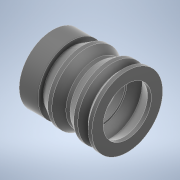
# Autodesk Inventor part: Daemper_TPU_Z2
Saved by Autodesk Inventor 2021 (Build 250183000, 183)
## iProperties
Created: 2022-06-20
Part Number: Daemper_TPU_Z2
Material: Thermoplastisches Harz
Document SubType Name: Modeling
Designer: Timo
Density: 1.28 g/cm^3
Appearance: Glatt - Schwarz
Mass: 1.13349 g
Surface Area: 19.2466 cm^2
Volume: 0.885539 cm^3
Author: Timo
Autodesk Inventor part; units mm, degrees
ref_plane "YZ Plane" through (0, 0, 0) normal (1, 0, 0) x (0, 1, 0)
ref_plane "XZ Plane" through (0, 0, 0) normal (0, 1, 0) x (-1, 0, 0)
ref_plane "XY Plane" through (0, 0, 0) normal (0, 0, 1) x (1, 0, 0)
sketch "Skizze1" plane through (0, 0, 0) normal (0, 0, 1) x (1, 0, 0)
  line L0 (-15, 0) -> (15, 0)
  line L1 (-5.5, 5.1) -> (-2.75, 6.7)
  line L2 (-2.75, 6.7) -> (0, 5.1)
  line L3 (0, 5.1) -> (2.75, 6.7)
  line L4 (2.75, 6.7) -> (5.5, 5.1)
  line L5 (-5.5, 5.1) -> (5.5, 5.1) construction
  line L6 (-2.75, 6.7) -> (2.75, 6.7) construction
  line L7 (0, 5.1) -> (5.5, 5.1) construction
  line L8 (5.5, 6.0256) -> (2.75, 7.6256)
  line L9 (2.75, 7.6256) -> (0, 6.0256)
  line L10 (0, 6.0256) -> (-2.75, 7.6256)
  line L11 (-2.75, 7.6256) -> (-5.5, 6.0256)
  line L12 (-5.5, 5.1) -> (-7.9, 5.1)
  line L13 (-7.9, 5.1) -> (-7.9, 3)
  line L14 (-7.9, 3) -> (-9.5, 3)
  line L15 (-9.5, 3) -> (-9.5, 7.1)
  line L16 (-9.5, 7.1) -> (-5.5, 7.1)
  line L17 (-5.5, 7.1) -> (-5.5, 6.0256)
  line L18 (5.5, 5.1) -> (5.5, 6.0256)
  line L19 (4.5639, 6.5702) -> (5.5, 7.5)
  line L20 (5.5, 7.5) -> (5.5, 6.0256)
  line L21 (5.5, 7.5) -> (6.3, 7.5)
  line L22 (6.3, 7.5) -> (6.3, 5.1)
  line L23 (6.3, 5.1) -> (5.5, 5.1)
  line L24 (5.5, 5.1) -> (5.5, 7.5)
  line L25 (-0.75, 5.1) -> (0.75, 5.1)
  line L26 (0.75, 5.1) -> (0.75, 5.5364)
  line L27 (0.75, 5.5364) -> (-0.75, 5.5364)
  line L28 (-0.75, 5.5364) -> (-0.75, 5.1)
  point P0 (0, 0)
  point P1 (0, 0)
  point P2 (0, 6.7)
  point P3 (2.75, 5.1)
  point P4 (0, 5.5364)
  point P5 (-0.75, 5.5364)
  dimension "d37" = 0.8
  dimension "d38" = 6
  dimension "d39" = 10.2
  dimension "d40" = 2
  dimension "d41" = 1.6
  dimension "d42" = 11
  dimension "d43" = 4
  dimension "d44" = 1.6
  dimension "d45" = 30
  dimension "d46" = 75
  dimension "d47" = 15
  dimension "d49" = 0.8
  dimension "d50" = 1.5
  constraints: 58 end point, 7 perpendicular, 7 vertical alignment, 6 horizontal, 5 midpoint, 4 parallel, 3 point on line, 2 collinear, 1 coincident, 1 vertical, 3 other
  measures "d37" distance between parallel lines of L1 L11
  measures "d38" diameter of L14 L0
  measures "d39" diameter of L12 L0
  measures "d40" distance between parallel lines of L16 L12
  measures "d41" distance from line of L5 L1.end
  measures "d42" distance of L8.start L11.end
  measures "d43" distance of L15.end L16.end
  measures "d44" distance of L13.end L14.end
  measures "d45" distance of L0.start L0.end
  measures "d46" angle of L19 L8
  measures "d47" diameter of L19.end L0
  measures "d49" distance of L22.end L4.end
  measures "d50" distance of L26.end L27.end
revolve "Umdrehung2" add sketch "Skizze1" angle 360 about axis through (-15, 0, 0) along (1, 0, 0)
chamfer "Fase3" distance 0.5 angle 45 3 edges at (-2.75, -7.6256, 0) (2.75, -7.6256, 0) (0, -6.0256, 0)
